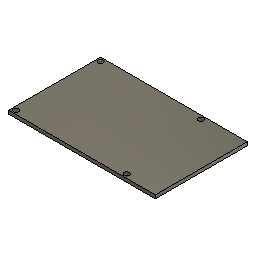
btt_pi_mount v15 (Autodesk Fusion 360 archive; units mm, degrees)
design "btt pi footprrint"
Autodesk Fusion 360 part; units mm, degrees
sketch "Sketch1" plane through (0, 0, 0) normal (0, 1, 0) x (1, 0, 0)
  line L0 (0, 0) -> (58, 0)
  line L1 (58, 0) -> (58, 49)
  line L2 (58, 49) -> (0, 49)
  line L3 (0, 49) -> (0, 0)
  line L4 (58, 0) -> (64, 0)
  circle A0 centre (0, 49) radius 1.5
  circle A1 centre (0, 0) radius 1.5
  circle A2 centre (64, 0) radius 1.5
  circle A3 centre (58, 49) radius 1.5
  line L5 (60.1599, -2.1599) -> (60.1599, 51.1599)
  line L6 (60.1599, 51.1599) -> (-2.1599, 51.1599)
  line L7 (-2.1599, 51.1599) -> (-2.1599, -2.1599)
  line L8 (-2.1599, -2.1599) -> (60.1599, -2.1599)
  line L9 (60.1599, 51.1599) -> (82.8401, 51.1599)
  line L10 (82.8401, 51.1599) -> (82.8401, -2.1599)
  line L11 (82.8401, -2.1599) -> (60.1599, -2.1599)
  line L12 (60.1599, -2.1599) -> (60.1599, 51.1599)
  dimension "d1" = 58
  dimension "d2" = 3
  dimension "d3" = 49
  dimension "d4" = 64
  dimension "d5" = 2.1599
  dimension "d6" = 85
  constraint horizontal L0
  constraint vertical L1
  constraint horizontal L2
  constraint vertical L3
  constraint coincident L0.start L3.end
  constraint perpendicular L1 L4
  constraint coincident L2.end L3.start
  constraint coincident L4.end A2.centre
  constraint coincident L1.end L2.start
  constraint equal A0 A3
  constraint equal A1 A3
  constraint equal A2 A3
  constraint horizontal L9
  constraint vertical L10
  constraint horizontal L11
  constraint vertical L12
  constraint collinear L8 L11
  measures "d1" distance of L1.end L2.end
  measures "d2" diameter of A1
  measures "d3" distance of L0.start L2.end
  measures "d4" distance of L0.start L4.end
  measures "d6" distance of L7 L10
extrude "Extrude1" add sketch "Sketch1" along normal blind 2 contours L0 L1 L2 L3 A0 A1 A3 | L5 L6 L7 L8 L12 | L5 L9 L10 L11 L12
